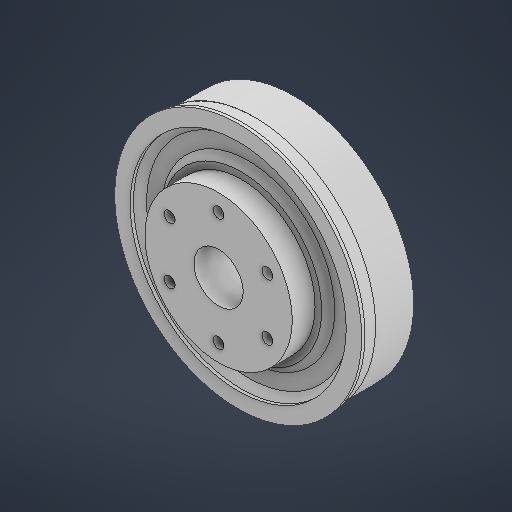
# Autodesk Inventor part: rotor_hub
Saved by Autodesk Inventor 2026.1 (Build 301233000, 233)
## iProperties
Created: 2025-03-04
Part Number: rotor_hub
Material: Generic
Document SubType Name: Modeling
Designer: aaron
Density: 1 g/cm^3
Appearance: Default
Author: aaron
Autodesk Inventor part; units mm, degrees
ref_plane "YZ Plane" through (0, 0, 0) normal (1, 0, 0) x (0, 1, 0)
ref_plane "XZ Plane" through (0, 0, 0) normal (0, 1, 0) x (-1, 0, 0)
ref_plane "XY Plane" through (0, 0, 0) normal (0, 0, 1) x (1, 0, 0)
sketch "Sketch1" plane through (0, 0, 0) normal (0, 0, 1) x (1, 0, 0)
  circle A0 centre (0, 0) radius 37
  dimension "d0" = 74
  constraints: 1 centre point, 1 coincident
  measures "d0" diameter of A0
extrude "Extrusion1" add sketch "Sketch1" along normal blind 22
sketch "Sketch2" plane through (0, 0, 22) normal (0, 0, 1) x (1, 0, 0)
  circle A0 centre (0, 0) radius 22.5
  dimension "d19" = 45
  constraints: 1 centre point, 1 coincident
  measures "d19" diameter of A0
extrude "Extrusion2" add sketch "Sketch2" along normal blind 7
sketch "Sketch7" plane through (0, 0, 22) normal (0, 0, 1) x (1, 0, 0)
  circle A0 centre (0, 0) radius 22.5 projected
  circle A1 centre (0, 0) radius 24.5
  circle A2 centre (0, 0) radius 37 projected
  circle A3 centre (0, 0) radius 33
  dimension "d12" = 2
  dimension "d13" = 4
  constraints: 2 centre point, 2 coincident
  measures "d12" radial gap between concentric circles of A0 A1
  measures "d13" radial gap between concentric circles of A3 A2
extrude "Extrusion5" cut sketch "Sketch7" against normal blind 2 contours A3
sketch "Sketch8" plane through (0, 0, 0) normal (0, 0, -1) x (-1, 0, 0)
  circle A0 centre (0, 0) radius 34
  circle A1 centre (0, 0) radius 37 projected
  dimension "d16" = 3
  constraints: 1 centre point, 1 coincident
  measures "d16" radial gap between concentric circles of A1 A0
extrude "Extrusion6" cut sketch "Sketch8" against normal blind 16 contours A0
sketch "Sketch9" plane through (0, 0, 29) normal (0, 0, 1) x (1, 0, 0)
  circle A0 centre (0, 0) radius 7.5
  dimension "d20" = 15
  constraints: 1 centre point, 1 coincident
  measures "d20" diameter of A0
extrude "Extrusion7" cut sketch "Sketch9" against normal blind 29
sketch "Sketch10" plane through (0, 0, 29) normal (0, 0, 1) x (1, 0, 0)
  circle A0 centre (0, 0) radius 17.25
  circle A1 centre (0, 17.25) radius 1.65
  circle A2 centre (-14.938938, 8.625) radius 1.65
  circle A3 centre (-14.938938, -8.625) radius 1.65
  circle A4 centre (0, -17.25) radius 1.65
  circle A5 centre (14.938938, -8.625) radius 1.65
  circle A6 centre (14.938938, 8.625) radius 1.65
  dimension "d23" = 34.5
  dimension "d24" = 3.3
  dimension "d27" = 360
  constraints: 6 centre point, 1 coincident, 1 vertical alignment, 15 other
  measures "d24" diameter of A1
extrude "Extrusion8" cut sketch "Sketch10" against normal through all contours A6 A0 | A0 A6 | A5 A0 | A0 A5 | A1 A0 | A0 A1 | A4 A0 | A0 A4 | A2 A0 | A0 A2 | A3 A0 | A0 A3
sketch "Sketch11" plane through (0, 0, 0) normal (0, 0, -1) x (-1, 0, 0)
  circle A0 centre (0, 0) radius 34 projected
  circle A1 centre (0, 0) radius 37 projected
extrude "Extrusion9" cut sketch "Sketch11" against normal blind 6
chamfer "Chamfer1" distance 4 angle 45 1 edges at (34, 0, 16)
sketch "Sketch12" plane through (0, 0, 22) normal (0, 0, 1) x (1, 0, 0)
  circle A0 centre (0, 0) radius 37 projected
  circle A1 centre (0, 0) radius 33 projected
  circle A2 centre (0, 0) radius 7.5 projected
  circle A3 centre (0, 0) radius 37.75
  dimension "d36" = 0.75
  constraints: 1 centre point, 1 coincident
  measures "d36" radial gap between concentric circles of A3 A0
extrude "Extrusion10" add sketch "Sketch12" along normal blind 1 contours A0 | A2 | A3
chamfer "Chamfer3" distance 2 angle 45 2 edges at (-33, 0, 20) (-24.5, 0, 20)
sketch "Sketch14" plane through (0, 0, 6) normal (0, 0, -1) x (-1, 0, 0)
  circle A0 centre (0, 0) radius 37 projected
  circle A1 centre (0, 0) radius 34 projected
  circle A2 centre (0, 0) radius 36.75
  dimension "d47" = 0.25
  constraints: 1 centre point
  measures "d47" radial gap between concentric circles of A0 A2
sketch "Sketch14 outline for Extrusion12" plane through (0, 0, 6) normal (0, 0, -1) x (-1, 0, 0)
  circle A0 centre (0, 0) radius 37
  circle A1 centre (0, 0) radius 36.75
extrude "Extrusion12" cut sketch "Sketch14 outline for Extrusion12" against normal blind 12
sketch "Sketch15" plane through (0, 0, 18) normal (0, 0, -1) x (-1, 0, 0)
  circle A0 centre (0, 0) radius 37 projected
  circle A1 centre (0, 0) radius 36.75 projected
  circle A2 centre (0, 0) radius 36.99
  dimension "d50" = 0.01
  constraints: 1 centre point
  measures "d50" radial gap between concentric circles of A0 A2
sketch "Sketch15 outline for Extrusion13" plane through (0, 0, 18) normal (0, 0, -1) x (-1, 0, 0)
  circle A0 centre (0, 0) radius 37
  circle A1 centre (0, 0) radius 36.99
extrude "Extrusion13" cut sketch "Sketch15 outline for Extrusion13" against normal up to surface (4 mm away)
sketch "Sketch16" plane through (0, 0, 6) normal (0, 0, -1) x (-1, 0, 0)
  circle A0 centre (0, 0) radius 36.75 projected
  circle A1 centre (0, 0) radius 34 projected
extrude "Extrusion14" cut sketch "Sketch16" against normal blind 0.1
sketch "Sketch17" plane through (0, 0, 29) normal (0, 0, 1) x (1, 0, 0)
  circle A0 centre (0, 0) radius 7.5 projected
extrude "Extrusion15" cut sketch "Sketch17" against normal through all
body "Solid1"
